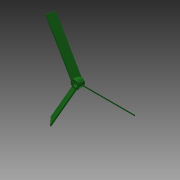
# Autodesk Inventor part: DAL T5040
Saved by Autodesk Inventor 2015 (Build 190159000, 159)
## iProperties
Created: 2016-11-27
Part Number: DAL T5040
Material: Generic
Document SubType Name: Modeling
Designer: Hampus
Density: 1 g/cm^3
Appearance: Smooth - Dark Forest Green
Author: Hampus
Autodesk Inventor part; units mm, degrees
ref_plane "YZ Plane" through (0, 0, 0) normal (1, 0, 0) x (0, 1, 0)
ref_plane "XZ Plane" through (0, 0, 0) normal (0, 1, 0) x (-1, 0, 0)
sketch "Sketch1" plane through (0, 0, 0) normal (0, 1, 0) x (-1, 0, 0)
  circle A0 centre (0, 0) radius 2.5
  circle A1 centre (0, 0) radius 63.5
  circle A2 centre (0, 0) radius 5
  dimension "d1" = 127
  dimension "d4" = 10
  constraints: 3 centre point, 3 coincident
  measures "d1" diameter of A1
  measures "d4" diameter of A2
extrude "Extrusion1" add sketch "Sketch1" along normal blind 7 contours A2
ref_plane "Work Plane1" through (5, 0, 0) normal (1, 0, 0) x (0, 1, 0)
sketch "Sketch3" plane through (5, 0, 0) normal (1, 0, 0) x (0, 1, 0)
  line L0 (7, -5) -> (7, 5) projected
  arc A0 (6.5749, -3.5929) -> (0.5749, 2.4071) centre (-24.5498, -28.7176) ccw
  line L1 (0.5749, 2.4071) -> (0.5749, 3.9071)
  arc A1 (0.5749, 3.9071) -> (6.5749, -2.0929) centre (22.8832, 20.2155) ccw
  line L2 (6.5749, -2.0929) -> (6.5749, -3.5929)
  point P0 (0, 0)
  dimension "d13" = 40
  dimension "d15" = 1.5
  constraints: 4 end point, 4 point on circle, 2 centre point, 2 vertical
  measures "d13" radius of A0
  measures "d15" distance of L1.start L1.end
extrude "Extrusion3" add sketch "Sketch3" against normal blind 2 and the other way blind 58.5
fillet "Fillet2" radius 0.25 4 edges at (5, 7, 0) (5, 0, 0) (2.5, 7, 0) (2.5, 0, 0)
pattern_circular "Circular Pattern1" count 3 over 360 about axis through (0, 0, 0) along (0, 1, 0) of "Extrusion3"
body "Solid1"
